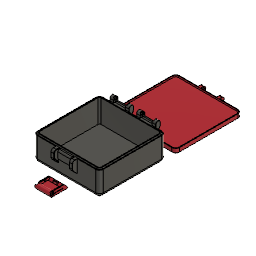
Milwaukee Tool Box Single Lock (Autodesk Fusion 360 design; units mm, degrees)
part number: 2025-08-27-12-33-30-467
Autodesk Fusion 360 part; units mm, degrees
sketch "Box" plane through (0, 0, 0) normal (0, 0, 1) x (1, 0, 0)
  line L0 (38, 43) -> (-38, 43)
  line L1 (-43, 38) -> (-43, -38)
  line L2 (-38, -43) -> (38, -43)
  line L3 (43, -38) -> (43, 38)
  line L4 (43, 43) -> (-43, -43) construction
  line L5 (-43, 43) -> (43, -43) construction
  arc A0 (-38, 43) -> (-43, 38) centre (-38, 38) ccw
  arc A1 (43, 38) -> (38, 43) centre (38, 38) ccw
  arc A2 (38, -43) -> (43, -38) centre (38, -38) ccw
  arc A3 (-43, -38) -> (-38, -43) centre (-38, -38) ccw
  line L6 (38, 40) -> (-38, 40)
  arc A4 (-38, 40) -> (-40, 38) centre (-38, 38) ccw
  line L7 (-40, 38) -> (-40, -38)
  arc A5 (-40, -38) -> (-38, -40) centre (-38, -38) ccw
  line L8 (-38, -40) -> (38, -40)
  arc A6 (38, -40) -> (40, -38) centre (38, -38) ccw
  line L9 (40, -38) -> (40, 38)
  arc A7 (40, 38) -> (38, 40) centre (38, 38) ccw
  line L10 (-41, 38) -> (-41, -38)
  arc A8 (-41, -38) -> (-38, -41) centre (-38, -38) ccw
  line L11 (-38, -41) -> (38, -41)
  arc A9 (38, -41) -> (41, -38) centre (38, -38) ccw
  line L12 (41, -38) -> (41, 38)
  arc A10 (41, 38) -> (38, 41) centre (38, 38) ccw
  line L13 (38, 41) -> (-38, 41)
  arc A11 (-38, 41) -> (-41, 38) centre (-38, 38) ccw
  dimension "d5" = 86
  dimension "d6" = 86
  dimension "d7" = 5
  dimension "d10" = -3
  dimension "d95" = 1
  constraint horizontal L0
  constraint perpendicular L0 L1
  constraint parallel L0 L2
  constraint parallel L1 L3
  constraint coincident L4 origin
  constraint coincident L5 origin
  constraint coincident L5.start L0
  constraint coincident L5.start L1
  constraint tangent L0 A0
  constraint tangent L1 A0
  constraint coincident L4.start L0
  constraint coincident L4.start L3
  constraint tangent L0 A1
  constraint tangent L3 A1
  constraint coincident L5.end L3
  constraint coincident L5.end L2
  constraint tangent L3 A2
  constraint tangent L2 A2
  constraint equal A1 A2
  constraint coincident L4.end L2
  constraint coincident L4.end L1
  constraint tangent L2 A3
  constraint tangent L1 A3
  constraint equal A0 A1
  constraint equal A0 A3
  measures "d5" distance of L4.end L5.end
  measures "d6" distance of L5.start L4.end
  measures "d7" radius of A0
extrude "Extrude1" add sketch "Box" along normal blind 31 contours L0 L1 L2 L3 A0 A1 A2 A3 makes body 1
extrude "Extrude15" add sketch "Box" along normal blind 32 contours L10 A8 L11 A9 L12 A10 L13 A11 bodies 1
extrude "Extrude2" add sketch "Box" along normal blind 2 contours L6 A4 L7 A5 L8 A6 L9 A7 bodies 1
chamfer "Chamfer7" distance 0.99 angle 45 8 edges at (0, -41, 31) (-40.1213, -40.1213, 31) (-41, 0, 31) (-40.1213, 40.1213, 31) (0, 41, 31) (40.1213, 40.1213, 31) (41, 0, 31) (40.1213, -40.1213, 31) on bodies 1
chamfer "Chamfer1" distance 3 angle 45 8 edges at (0, -43, 0) (41.5355, -41.5355, 0) (43, 0, 0) (41.5355, 41.5355, 0) (0, 43, 0) (-41.5355, 41.5355, 0) (-43, 0, 0) (-41.5355, -41.5355, 0) on bodies 1
fillet "Fillet1" radius 4 8 edges at (-41.5355, 41.5355, 3) (0, 43, 3) (41.5355, 41.5355, 3) (43, 0, 3) (41.5355, -41.5355, 3) (0, -43, 3) (-41.5355, -41.5355, 3) (-43, 0, 3) on bodies 1
sketch "Lid" plane through (0, 0, 31) normal (0, 0, 1) x (-1, 0, 0)
  arc A0 (43, 38) -> (38, 43) centre (38, 38) ccw
  line L0 (38, 43) -> (-38, 43)
  arc A1 (-38, 43) -> (-43, 38) centre (-38, 38) ccw
  line L1 (-43, 38) -> (-43, -38)
  arc A2 (-43, -38) -> (-38, -43) centre (-38, -38) ccw
  line L2 (-38, -43) -> (38, -43)
  arc A3 (38, -43) -> (43, -38) centre (38, -38) ccw
  line L3 (43, -38) -> (43, 38)
  arc A4 (38, -43) -> (43, -38) centre (38, -38) ccw
  line L4 (-38, -43) -> (38, -43)
  line L5 (43, -38) -> (43, 38)
  arc A5 (43, 38) -> (38, 43) centre (38, 38) ccw
  line L6 (38, 43) -> (-38, 43)
  arc A6 (-38, 43) -> (-43, 38) centre (-38, 38) ccw
  line L7 (-43, 38) -> (-43, -38)
  arc A7 (-43, -38) -> (-38, -43) centre (-38, -38) ccw
  line L8 (42.1, -38) -> (42.1, 38)
  arc A8 (42.1, 38) -> (38, 42.1) centre (38, 38) ccw
  line L9 (38, 42.1) -> (-38, 42.1)
  arc A9 (-38, 42.1) -> (-42.1, 38) centre (-38, 38) ccw
  line L10 (-42.1, 38) -> (-42.1, -38)
  arc A10 (-42.1, -38) -> (-38, -42.1) centre (-38, -38) ccw
  line L11 (-38, -42.1) -> (38, -42.1)
  arc A11 (38, -42.1) -> (42.1, -38) centre (38, -38) ccw
  arc A12 (-41.99, -38) -> (-38, -41.99) centre (-38, -38) ccw
  dimension "d18" = -0.9
extrude "Extrude3" add sketch "Lid" along normal blind 6 separate body contours A0 L0 A1 L1 A2 L2 A3 L3 A4 L4 L5 A5 L6 A6 L7 A7 | L8 A8 L9 A9 L10 A10 L11 A11 makes body 2
extrude "Extrude16" cut sketch "Lid" along normal blind 1 contours L8 A8 L9 A9 L10 A10 L11 A11 bodies 2
chamfer "Chamfer8" distance 1 angle 45 16 edges at (-40.8991, 40.8991, 32) (-42.1, 0, 32) (-40.8991, -40.8991, 32) (0, -42.1, 32) (40.8991, -40.8991, 32) (42.1, 0, 32) (40.8991, 40.8991, 32) (0, 42.1, 32) (0, -43, 37) (41.5355, -41.5355, 37) (43, 0, 37) (41.5355, 41.5355, 37) (0, 43, 37) (-41.5355, 41.5355, 37) (-43, 0, 37) (-41.5355, -41.5355, 37) on bodies 2
sketch "Lid Hinge and Latch" plane through (0, 0, 0) normal (1, 0, 0) x (0, 1, 0)
  circle A0 centre (46.2, 34) radius 1.8
  line L0 (43, 31) -> (46.2, 31)
  circle A1 centre (-46.2, 34) radius 1.8 construction
  line L1 (-44.8771, 32.5) -> (-43.9639, 32)
  circle A2 centre (-46.2, 34) radius 2
  circle A3 centre (-46.2, 34) radius 3
  line L2 (-44.8771, 35.5) -> (-43.9639, 36)
  line L3 (-49.2, 34) -> (-49.2, 14)
  line L4 (-49.2, 14) -> (-47.7, 14)
  line L5 (-47.7, 14) -> (-43, 18.7)
  line L6 (-43, 18.7) -> (-43, 31.4722)
  line L7 (-46.5, 31.015) -> (-46.5, 20.7)
  line L8 (-46.5, 20.7) -> (-43.5, 20.7)
  line L9 (-46, 20.7) -> (-46, 31.0067)
  line L10 (-43.9639, 32) -> (-43, 31.4722)
  line L11 (-43.5, 20.7) -> (-43, 20.2)
  line L12 (-46.5, 20.7) -> (-43.75, 17.95)
  line L13 (43, 31) -> (43, 36)
  line L14 (-43, 4.6569) -> (-43, 31)
  line L15 (43, 4.6569) -> (43, 31)
  line L16 (-49.2, 34) -> (-49.2, 35.2426)
  line L17 (-49.2, 35.2426) -> (-48.3213, 36.1213)
  line L18 (-38, 0) -> (-40, 0)
  line L19 (42, 37) -> (47, 37)
  line L20 (47, 37) -> (47.6938, 36.6017)
  line L21 (43, 36) -> (42, 37)
  circle A4 centre (46.2, 34) radius 3
  line L22 (-43, 31) -> (-43, 36)
  point P0 (-43, 31.4722)
  point P1 (-38, 0)
  point P2 (42, 37)
  dimension "d37" = 3.6
  dimension "d110" = 3.6
  dimension "d111" = 6
  dimension "d112" = 4
  dimension "d113" = 4
  dimension "d114" = 3
  dimension "d120" = 45
  dimension "d121" = 1.5
  dimension "d124" = 3
  dimension "d130" = 0.5
  dimension "d131" = 2
  dimension "d132" = 45
  dimension "d133" = 0.5
  dimension "d277" = 1.2426
  dimension "d337" = 89.2
  dimension "d342" = 34
  dimension "d343" = 14
  dimension "d353" = 5
  dimension "d354" = 29.863
  dimension "d355" = 6
  dimension "d356" = 89.2
  constraint coincident L1.end A3
  constraint coincident L2.end A3
  constraint concentric A1 A2
  constraint coincident L1.start A2
  constraint coincident A1.centre A2.centre
  constraint coincident L2.start A2
  constraint vertical L1.start L2.start
  constraint vertical L2.end L1.end
  constraint vertical L3
  constraint tangent A3 L3
  constraint perpendicular L3 L4
  constraint perpendicular L4 L6
  constraint vertical L7
  constraint vertical L9
  constraint parallel L1 L10
  constraint coincident A3 L7.start
  constraint coincident A3 L9.end
  constraint horizontal L8
  constraint coincident L9.start L8
  constraint coincident L6 L11.end
  constraint coincident L5 L12.end
  constraint perpendicular L5 L12
  constraint coincident A3 L3.start
  constraint coincident P0 L6.end
  constraint coincident P0 L14
  constraint coincident L0.start L13.start
  constraint perpendicular L0 L13
  constraint parallel L3 L16
  constraint coincident A3 L17.end
  constraint coincident L3.start L16.start
  constraint tangent A3 L17
  constraint horizontal L19
  constraint coincident P2 L19.start
  constraint concentric A0 A4
  constraint coincident L0.end A4
  constraint tangent L0 A4
  constraint coincident L20.end A4
  constraint tangent L20 A4
  measures "d37" diameter of A0
  measures "d110" diameter of A1
  measures "d111" diameter of A3
  measures "d112" distance of L2.end L1.end
  measures "d113" diameter of A2
  measures "d114" distance of L1.start L2.start
  measures "d120" angle of L4 L5
  measures "d121" distance of L3.end L4.end
  measures "d124" distance of L6 L9
  measures "d130" distance of L7.end L9.start
  measures "d131" distance of L5.end L8
  measures "d132" angle of L6 L11
  measures "d133" distance of L6 L8.end
  measures "d277" distance of L3.start L16.end
  measures "d337" distance of A1.centre L15
  measures "d342" distance of A1.centre L18
  measures "d343" distance of L4 L18
  measures "d353" distance of P2 L19.end
  measures "d354" angle of L19 L20
  measures "d355" diameter of A4
  measures "d356" distance of A0.centre L22
extrude "Extrude7" add sketch "Lid Hinge and Latch" along normal mid plane 15 from surface at 17.3333 separate body contours L0 L13 L19 L21 A4 | A4 | L19 L20 A4 makes body 3
extrude "Extrude8" add sketch "Lid Hinge and Latch" along normal mid plane 18 from surface at 17.3333 contours A0 bodies 3
chamfer "Chamfer2" distance 0.5 angle 45 2 faces at (8.3333, 46.7552, 33.4017) (26.3333, 46.7552, 33.4017) on bodies 3
sketch "Lid Hinge Cut" plane through (0, 43, 0) normal (0, 1, 0) x (-1, 0, 0)
  line L0 (-38, 31) -> (38, 31)
  line L1 (38, 31) -> (38, 36)
  line L2 (-38, 36) -> (-38, 31)
  line L3 (-24.8333, 35.8) -> (-26.3333, 34.934) construction
  line L4 (-26.3333, 34.934) -> (-26.3333, 35.8) construction
  line L5 (-26.3333, 35.8) -> (-24.8333, 35.8) construction
  line L6 (-9.8333, 35.8) -> (-8.3333, 34.934) construction
  line L7 (-8.3333, 34.934) -> (-8.3333, 35.8) construction
  line L8 (-8.3333, 35.8) -> (-9.8333, 35.8) construction
  line L9 (-25.8333, 35.8) -> (-25.8333, 32.2)
  line L10 (-8.8333, 32.2) -> (-8.8333, 35.8)
  line L11 (-26.3333, 32.7) -> (-26.3333, 35.3)
  line L12 (-8.3333, 35.3) -> (-8.3333, 32.7)
  line L13 (38, 36) -> (-38, 36)
  line L14 (-9.8333, 31) -> (-9.8333, 36)
  line L15 (-24.8333, 36) -> (-24.8333, 31)
  line L16 (-19.8333, 37) -> (-14.8333, 37)
  line L17 (-14.8333, 37) -> (-14.8333, 31)
  line L18 (-14.8333, 31) -> (-19.8333, 31)
  line L19 (-19.8333, 31) -> (-19.8333, 37)
  line L20 (-9.8333, 37) -> (-24.8333, 37)
  dimension "d357" = 30
  dimension "d358" = 30
  dimension "d365" = 5
  dimension "d366" = 5
  constraint perpendicular L0 L4
  constraint perpendicular L4 L5
  constraint perpendicular L0 L7
  constraint perpendicular L7 L8
  constraint coincident L3.end L11
  constraint coincident L6.end L12
  constraint coincident L3.start L15
  constraint coincident L6.start L14
  constraint coincident L5 L9.start
  constraint coincident L8 L10.end
  constraint horizontal L16
  constraint vertical L17
  constraint horizontal L18
  constraint vertical L19
  constraint coincident L0 L17.end
  constraint coincident L16.start L20
  measures "d357" angle of L3 L5
  measures "d358" angle of L6 L8
  measures "d365" distance of L17 L20.start
  measures "d366" distance of L16.start L20.end
extrude "Extrude40" cut sketch "Lid Hinge Cut" along normal through all contours L0 L13 L17 L18 L19 | L13 L16 L17 L19 L20 bodies 3
extrude "Extrude26" add sketch "Lid Hinge and Latch" along normal mid plane 20 separate body contours L1 A2 A3 L2 | A3 L6 L8 L9 L10 L11 L14 L22 | A3 L3 L4 L5 L7 L12 | L5 L6 L8 L11 L12 L14 | A3 L16 L17 picked at (-44.3747, 35.9359) makes body 4
extrude "Extrude27" add sketch "Lid Hinge and Latch" along normal mid plane 17 contours A2 bodies 4
extrude "Extrude28" add sketch "Lid Hinge and Latch" along normal mid plane 18 contours L1 A2 A3 L2 picked at (-44.1133, 35.6507) bodies 4
chamfer "Chamfer14" distance 0.49 angle 45 2 edges at (8.5, -48.0647, 34.7232) (-8.5, -48.0647, 34.7232) on bodies 4
chamfer "Chamfer15" distance 0.5 angle 45 2 edges at (9, -43.2, 34) (-9, -43.2, 34) on bodies 4
extrude "Extrude29" cut sketch "Lid Hinge and Latch" along normal mid plane 17 contours A3 L6 L8 L9 L10 L11 L14 L22 | L5 L6 L8 L11 L12 L14 bodies 4
extrude "Extrude30" add sketch "Lid Hinge and Latch" along normal mid plane 5 contours L5 L6 L8 L11 L12 L14 bodies 4
chamfer "Chamfer18" distance 0.4 angle 45 3 edges at (8.5, -43, 25.0861) (-8.5, -43, 25.0861) (0, -49.2, 14) on bodies 4
fillet "Fillet4" radius 1 1 edges at (0, -47.7, 14) on bodies 4
sketch "Box and Lacth Hinge" plane through (0, 0, 0) normal (1, 0, 0) x (0, 1, 0)
  line L0 (43, 31) -> (43, 23)
  line L1 (-46.2, 37) -> (-42, 37)
  line L2 (-46, 29) -> (-46, 21.2)
  line L3 (-45.5, 20.7) -> (-43, 20.7)
  line L4 (-43, 14) -> (-43, 31)
  line L5 (-46, 21.2) -> (-45.5, 20.7)
  arc A0 (-46.2, 31) -> (-49.2, 28) centre (-46.2, 28) ccw
  line L6 (-49.2, 28) -> (-49.2, 21.8569)
  line L7 (-48.0284, 19.0284) -> (-43, 14)
  line L8 (-45.5, 20.7) -> (-43, 18.2)
  line L9 (43.2, 31) -> (43.2, 34)
  line L10 (48.0284, 28.0284) -> (43, 23)
  arc A1 (-49.2, 21.8569) -> (-48.0284, 19.0284) centre (-45.2, 21.8569) ccw
  circle A2 centre (-46.2, 34) radius 3
  line L11 (-43, 31) -> (-46.2, 31)
  arc A3 (-44, 31) -> (-46, 29) centre (-44, 29) ccw
  line L12 (43, 31) -> (45.0864, 31)
  line L13 (-43, 31) -> (-43, 36)
  circle A4 centre (-46.2, 34) radius 1.8
  arc A5 (48.0284, 28.0284) -> (49.2, 30.8569) centre (45.2, 30.8569) ccw
  line L14 (49.2, 34) -> (49.2, 30.8569)
  circle A6 centre (46.2, 34) radius 2
  circle A7 centre (46.2, 34) radius 1.8 construction
  circle A8 centre (46.2, 34) radius 3
  line L15 (47.7, 35.3229) -> (48.2, 36.2361)
  line L16 (44.7, 35.3229) -> (44.2, 36.2361)
  circle A9 centre (46.2, 34) radius 3.2 construction
  line L17 (43, 31) -> (46.2, 31)
  line L18 (-38, 0) -> (38, 0)
  line L19 (-43, 36) -> (-42, 37)
  line L20 (-46.2, 37) -> (-47, 37)
  line L21 (-47, 37) -> (-47.6938, 36.6017)
  circle A10 centre (46.2, 34) radius 1.3
  line L22 (47.3136, 31) -> (49.2, 31)
  arc A11 (45.0864, 31) -> (47.3136, 31) centre (46.2, 34) ccw
  point P0 (-46, 20.7)
  point P1 (-46, 20.7)
  point P2 (-49.2, 34)
  point P3 (-48.8, 14)
  point P4 (43, 31)
  point P5 (43, 31)
  point P6 (43, 36)
  dimension "d136" = 0.5
  dimension "d137" = 0.5
  dimension "d140" = 3
  dimension "d150" = 45
  dimension "d182" = 45
  dimension "d239" = 4
  dimension "d244" = 3
  dimension "d252" = 2
  dimension "d270" = 4
  dimension "d309" = 3.6
  dimension "d310" = 6
  dimension "d311" = 4
  dimension "d312" = 4
  dimension "d313" = 3
  dimension "d321" = 6.4
  dimension "d352" = 23
  dimension "d363" = 0.8
  constraint vertical L2
  constraint horizontal L3
  constraint vertical L4
  constraint coincident P1 L2
  constraint coincident P1 L3
  constraint horizontal A0.end A0.centre
  constraint vertical L6
  constraint parallel L5 L8
  constraint coincident L4 L3.end
  constraint vertical L9
  constraint coincident L0.end L10.end
  constraint vertical L0
  constraint tangent L6 A1
  constraint tangent L7 A1
  constraint coincident A2 A0.start
  constraint tangent A2 L11
  constraint horizontal L11
  constraint coincident L11 A3.start
  constraint tangent L2 A3
  constraint tangent L11 A3
  constraint coincident P1 P0
  constraint coincident L4 L8.end
  constraint vertical A0.end P2
  constraint coincident L1.start A2
  constraint horizontal L1
  constraint horizontal L4.start P3
  constraint horizontal L12
  constraint coincident P5 P4
  constraint coincident L12 A11.start
  constraint tangent L10 A5
  constraint vertical L14
  constraint coincident A5.end L14.end
  constraint tangent A5 L14
  constraint coincident L15.end A8
  constraint coincident L16.end A8
  constraint concentric A6 A7
  constraint coincident L15.start A6
  constraint coincident L16.start A6
  constraint coincident L9.end A8
  constraint horizontal L9.end A6.centre
  constraint coincident L14.start A8
  constraint concentric A8 A9
  constraint horizontal L14.start A6.centre
  constraint horizontal L15.start L16.start
  constraint horizontal L16.end L15.end
  constraint vertical L1.start A2.centre
  constraint coincident A6.centre A7.centre
  constraint coincident L12 L9.start
  constraint tangent A2 L20
  constraint coincident A2 L21.end
  constraint tangent A2 L21
  constraint coincident L1.end L19.end
  constraint coincident A9 L22.start
  constraint coincident L14 L22.end
  constraint perpendicular L14 L22
  constraint horizontal L12.end L22.start
  constraint coincident L12.end A9
  constraint concentric A9 A11
  measures "d136" distance of P1 L2.end
  measures "d137" distance of P1 L3.start
  measures "d140" distance of L2 L4
  measures "d150" angle of L4 L7
  measures "d182" angle of L0 L10
  measures "d239" radius of A1
  measures "d244" radius of A0
  measures "d252" radius of A3
  measures "d270" radius of A5
  measures "d309" diameter of A7
  measures "d310" diameter of A8
  measures "d311" distance of L16.end L15.end
  measures "d312" diameter of A6
  measures "d313" distance of L15.start L16.start
  measures "d321" diameter of A9
  measures "d352" distance of L0.end L18
  measures "d363" distance of L1.start L20.end
extrude "Extrude11" add sketch "Box and Lacth Hinge" along normal mid plane 25 from surface at 17.3333 separate body contours L0 L10 L12 A5 L14 L17 L22 A11 | L9 L12 A8 L17 | A6 A8 L15 L16 | L14 A8 L17 L22 A11 | A6 A8 L15 L16 | A6 | A10 makes body 5
extrude "Extrude10" cut sketch "Box and Lacth Hinge" along normal mid plane 15.4 from surface at 17.3333 contours L9 L12 A8 L17 | A6 A8 L15 L16 | L14 A8 L17 L22 A11 | A6 A8 L15 L16 | L1 A2 L11 L13 L19 bodies 5
extrude "Extrude12" cut sketch "Box and Lacth Hinge" along normal mid plane 18.4 from surface at 17.3333 contours A6 | A10 bodies 5
extrude "Extrude39" cut sketch "Box and Lacth Hinge" along normal mid plane 17.4 from surface at 17.3333 contours A6 A8 L15 L16 picked at (44.5493, 36.0867) bodies 5
chamfer "Chamfer4" distance 0.499 angle 45 2 faces at (8.1333, 45.0225, 34.3325) (26.5333, 45.0225, 33.754) on bodies 5
chamfer "Chamfer21" distance 0.5 distance2 0.5 2 edges at (8.6333, 46.2, 37) (26.0333, 46.2, 37) measured on face at (6.4333, 43.8719, 35.892) measured on face at (28.2333, 43.8719, 35.892) on bodies 5
chamfer "Chamfer3" distance 0.2 angle 45 10 edges at (4.8333, 46.2, 37) (4.8333, 49.2, 32.4284) (4.8333, 48.8955, 29.3261) (4.8333, 45.5142, 25.5142) (4.8333, 43.2, 32.5) (29.8333, 49.2, 32.4284) (29.8333, 46.2, 37) (29.8333, 43.2, 32.5) (29.8333, 45.5142, 25.5142) (29.8333, 48.8955, 29.3261) on bodies 5
extrude "Extrude31" add sketch "Box and Lacth Hinge" along normal mid plane 28 contours L1 A2 L11 L13 L19 | A2 | A2 L20 L21 | A4 bodies 2
extrude "Extrude32" cut sketch "Box and Lacth Hinge" along normal mid plane 20.4 contours L1 A2 L11 L13 L19 | A2 | A2 L20 L21 bodies 2
extrude "Extrude33" cut sketch "Box and Lacth Hinge" along normal mid plane 17.4 contours A4 bodies 2
chamfer "Chamfer17" distance 0.5 angle 45 2 edges at (8.7, -47.8782, 33.3491) (-8.7, -47.8782, 34.6509) on bodies 2
chamfer "Chamfer16" distance 0.2 angle 45 6 edges at (14, -49.0987, 33.227) (14, -47.3469, 36.8008) (14, -44.6, 31) (-14, -49.0987, 33.227) (-14, -44.6, 31) (-14, -47.3469, 36.8008) on bodies 2
extrude "Extrude21" add sketch "Box and Lacth Hinge" along normal mid plane 28 separate body contours L2 L4 L5 A0 L6 L7 L8 A1 L11 A3 | L2 L3 L4 L5 L11 A3 | L3 L4 L8 makes body 6
extrude "Extrude22" cut sketch "Box and Lacth Hinge" along normal mid plane 20.4 contours L2 L4 L5 A0 L6 L7 L8 A1 L11 A3 | L2 L3 L4 L5 L11 A3 | L3 L4 L8 bodies 6 makes body 7 at (14, -44.6761, 21.3428)
chamfer "Chamfer11" distance 0.2 angle 45 10 edges at (-14, -49.2, 24.9284) (-14, -48.3213, 30.1213) (-14, -44.6, 31) (-14, -45.5142, 16.5142) (-14, -48.8955, 20.3261) (14, -49.2, 24.9284) (14, -48.8955, 20.3261) (14, -45.5142, 16.5142) (14, -44.6, 31) (14, -48.3213, 30.1213) on bodies 6 7
sketch "Latch Side" plane through (0, 0, 0) normal (1, 0, 0) x (0, 1, 0)
  line L0 (-48.0284, 19.0284) -> (-43, 14)
  line L1 (-43, 14) -> (-43, 31)
  arc A0 (-46.2, 31) -> (-49.2, 28) centre (-46.2, 28) ccw
  line L2 (-49.2, 28) -> (-49.2, 21.8569)
  arc A1 (-49.2, 21.8569) -> (-48.0284, 19.0284) centre (-45.2, 21.8569) ccw
  line L3 (-43, 31) -> (-46.2, 31)
  line L4 (-43, 30) -> (-46.2, 30)
  arc A2 (-46.2, 30) -> (-48.2, 28) centre (-46.2, 28) ccw
  line L5 (-48.2, 28) -> (-48.2, 21.8569)
  arc A3 (-48.2, 21.8569) -> (-47.3213, 19.7355) centre (-45.2, 21.8569) ccw
  line L6 (-47.3213, 19.7355) -> (-43, 15.4142)
  dimension "d224" = -1
  constraint coincident L1 L6.end
  constraint coincident L1 L4.start
extrude "Extrude25" cut sketch "Latch Side" along normal mid plane 21.4 contours L1 L4 A2 L5 A3 L6 bodies 6 7
chamfer "Chamfer13" distance 0.49 angle 45 10 edges at (-10.7, -44.6, 30) (-10.7, -45.1607, 17.5749) (-10.7, -47.9716, 20.7088) (-10.7, -48.2, 24.9284) (-10.7, -47.6142, 29.4142) (10.7, -47.6142, 29.4142) (10.7, -48.2, 24.9284) (10.7, -47.9716, 20.7088) (10.7, -45.1607, 17.5749) (10.7, -44.6, 30) on bodies 6 7
extrude "Extrude19" add sketch "Box and Lacth Hinge" along normal mid plane 16.6 separate body contours L2 L3 L4 L5 L11 A3 | L3 L4 L8 makes body 8
extrude "Extrude20" cut sketch "Box and Lacth Hinge" along normal mid plane 5.6 contours L3 L4 L8 bodies 8
ref_plane "WorkPlane1" through (0, -44.5, 24.6) normal (0, 1, 0) x (0, 0, 1)
sketch "Nub" plane through (0, -44.5, 0) normal (0, 1, 0) x (1, 0, 0)
  line L0 (-8.3, -25.1) -> (8.3, -25.1)
  line L1 (-8.3, -21.2) -> (-8.3, -29)
  line L2 (8.3, -29) -> (8.3, -21.2)
  line L3 (-8.3, -25.1) -> (-8.9, -25.1)
  line L4 (-7.9, -26.1) -> (7.9, -26.1)
  line L5 (8.3, -25.1) -> (8.9, -25.1)
  line L6 (-8.9, -25.1) -> (8.9, -25.1)
  arc A0 (-8.9, -25.1) -> (-7.9, -26.1) centre (-7.9, -25.1) ccw
  arc A1 (7.9, -26.1) -> (8.9, -25.1) centre (7.9, -25.1) ccw
  arc A2 (-9.015, -25.1) -> (-7.9, -26.215) centre (-7.9, -25.1) ccw
  line L7 (-7.9, -26.215) -> (7.9, -26.215)
  arc A3 (7.9, -26.215) -> (9.015, -25.1) centre (7.9, -25.1) ccw
  line L8 (-9.015, -25.1) -> (-8.9, -25.1)
  line L9 (8.9, -25.1) -> (9.015, -25.1)
  point P0 (0, -25.1)
  dimension "d176" = 1
  dimension "d225" = 16.6
  dimension "d226" = 17.8
  dimension "d228" = 1
  dimension "d229" = 1
  dimension "d231" = 0.115
  constraint horizontal L0
  constraint coincident L0.end L2
  constraint midpoint L0.start L1
  constraint perpendicular L1 L3
  constraint perpendicular L2 L4
  constraint horizontal L5
  constraint equal L3 L5
  constraint midpoint L0 P0
  constraint midpoint P0 L6
  constraint tangent L4 A0
  constraint coincident L3.end L6.start
  constraint tangent L4 A1
  constraint parallel L3 L8
  constraint parallel L5 L9
  measures "d176" distance of L0 L4
  measures "d225" distance of L0.start L0.end
  measures "d226" distance of L3.end L5.end
  measures "d228" radius of A0
  measures "d229" radius of A1
revolve "Revolve1" add sketch "Nub" angle 360 about axis through (-8.3, -44.5, 25.1) along (1, 0, 0) contours L0 L1 L2 L4 L6 A0 A1 | L1 L3 L6 A0 | L2 L5 L6 A1 bodies 8
revolve "Revolve2" cut sketch "Nub" angle 360 about axis through (-8.3, -44.5, 25.1) along (1, 0, 0) contours L1 L3 L6 A0 | L2 L5 L6 A1 | L1 A0 A2 L8 | L2 A1 A3 L9 bodies 4
mirror "Mirror8" about plane through (0, 0, 0) normal (1, 0, 0) of bodies 3 5 makes body 9 at (-13.2333, 43, 28.3333) makes body 10 at (-23.1667, 44, 37)
combine "Combine8" operation add target body 2 tool bodies 3 10
combine "Combine9" operation add target body 1 tool bodies 6 7 5 9 8
sketch "Column Divider" plane through (0, 0, 2) normal (0, 0, 1) x (-1, 0, 0)
  arc A0 (-40, -38) -> (-38, -40) centre (-38, -38) ccw
  line L0 (-38, -40) -> (38, -40)
  arc A1 (38, -40) -> (40, -38) centre (38, -38) ccw
  line L1 (40, -38) -> (40, 38)
  arc A2 (40, 38) -> (38, 40) centre (38, 38) ccw
  line L2 (38, 40) -> (-38, 40)
  arc A3 (-38, 40) -> (-40, 38) centre (-38, 38) ccw
  line L3 (-40, 38) -> (-40, -38)
  line L4 (41, -41) -> (41, 41)
  line L5 (40, 1) -> (42, 1)
  line L6 (42, 1) -> (42, -1)
  line L7 (42, -1) -> (40, -1)
  line L8 (40, -1) -> (40, 1)
  line L9 (40, 1) -> (42, -1) construction
  line L10 (42, 1) -> (40, -1) construction
  point P0 (38, 41)
  point P1 (41, 38)
  point P2 (38, -41)
  point P3 (41, -38)
  point P4 (41, 0)
  dimension "d344" = 2
  dimension "d345" = 2
  constraint vertical L4
  constraint horizontal L4.start P2
  constraint horizontal L4.end P0
  constraint coincident L4 P1
  constraint horizontal L5
  constraint perpendicular L5 L6
  constraint parallel L5 L7
  constraint parallel L6 L8
  constraint coincident L9 P4
  constraint coincident L10 P4
  constraint midpoint L4 P4
  measures "d344" distance of L6.end L7.end
  measures "d345" distance of L5.end L6.end
extrude "Extrude35" add sketch "Column Divider" along normal blind 30 thin wall 2 centred separate body open curves L4 makes body 11
extrude "Extrude41" add sketch "Column Divider" against normal blind 2 contours L1 L4 L5 L7 L8 | L4 L5 L6 L7 bodies 11
pattern_linear "R-Pattern1" count 1 spacing 82 along (1, 0, 0) of bodies 11 merged
delete_body "RemoveBody1" bodies 11
sketch "Row Divider" plane through (0, 0, 2) normal (0, 0, 1) x (-1, 0, 0)
  arc A0 (-40, -38) -> (-38, -40) centre (-38, -38) ccw
  line L0 (-38, -40) -> (38, -40)
  arc A1 (38, -40) -> (40, -38) centre (38, -38) ccw
  line L1 (40, -38) -> (40, 38)
  arc A2 (40, 38) -> (38, 40) centre (38, 38) ccw
  line L2 (38, 40) -> (-38, 40)
  arc A3 (-38, 40) -> (-40, 38) centre (-38, 38) ccw
  line L3 (-40, 38) -> (-40, -38)
  line L4 (41, 41) -> (-41, 41)
  line L5 (-1, 42) -> (1, 42)
  line L6 (1, 42) -> (1, 40)
  line L7 (1, 40) -> (-1, 40)
  line L8 (-1, 40) -> (-1, 42)
  line L9 (-1, 42) -> (1, 40) construction
  line L10 (1, 42) -> (-1, 40) construction
  point P0 (38, 41)
  point P1 (41, 38)
  point P2 (-41, 38)
  point P3 (0, 41)
  dimension "d348" = 2
  dimension "d349" = 2
  constraint horizontal L4
  constraint coincident L4 P0
  constraint vertical L4.start P1
  constraint vertical L4.end P2
  constraint horizontal L5
  constraint perpendicular L5 L6
  constraint parallel L5 L7
  constraint parallel L6 L8
  constraint coincident L9 P3
  constraint coincident L10 P3
  constraint midpoint L4 P3
  measures "d348" distance of L6.end L7.end
  measures "d349" distance of L5.end L6.end
extrude "Extrude36" add sketch "Row Divider" along normal blind 30 thin wall 2 centred separate body open curves L4 makes body 12
extrude "Extrude42" add sketch "Row Divider" against normal blind 2 contours L2 L4 L6 L7 L8 | L4 L5 L6 L8 bodies 12
pattern_linear "R-Pattern2" count 1 spacing 82 along (0, 1, 0) of bodies 12 merged
delete_body "RemoveBody2" bodies 12
sketch "Sketch20" plane through (0, 0, 37) normal (0, 0, 1) x (-1, 0, 0)
  line L0 (-14, 42) -> (-38, 42)
  arc A0 (-38, 42) -> (-42, 38) centre (-38, 38) ccw
  line L1 (-42, 38) -> (-42, -38)
  arc A1 (-42, -38) -> (-38, -42) centre (-38, -38) ccw
  arc A2 (38, -42) -> (42, -38) centre (38, -38) ccw
  line L2 (42, -38) -> (42, 38)
  arc A3 (42, 38) -> (38, 42) centre (38, 38) ccw
  line L3 (-25, -43) -> (25, -43) construction
  line L4 (25, -43) -> (25, 43) construction
  line L5 (25, 43) -> (-25, 43) construction
  line L6 (-25, 43) -> (-25, -43) construction
  line L7 (-25, -43) -> (25, 43) construction
  line L8 (25, -43) -> (-25, 43) construction
  line L9 (-26.1621, -4.1639) -> (-12.9321, 0.866)
  line L10 (-12.9321, 0.866) -> (-13.6937, -0.7988)
  line L11 (-13.6937, -0.7988) -> (4.2298, 5.3292)
  line L12 (4.2298, 5.3292) -> (3.238, 3.2747)
  line L13 (3.238, 3.2747) -> (24.0483, 11.2623)
  line L14 (24.0483, 11.2623) -> (8.4096, 7.3482)
  line L15 (8.4096, 7.3482) -> (9.7025, 9.8101)
  line L16 (9.7025, 9.8101) -> (-9.6733, 2.6017)
  line L17 (-9.6733, 2.6017) -> (-8.5752, 4.7447)
  line L18 (-8.5752, 4.7447) -> (-26.1621, -4.1639)
  line L19 (12.3768, -8.1134) -> (14.6615, -6.1829)
  spline S0 degree 2 poles (14.6615, -6.1829) (15.5648, -7.2101) (15.6533, -7.281) knots 0 0 0 1 1 1
  spline S1 degree 2 poles (15.6533, -7.281) (15.7242, -7.2101) (17.6015, -5.6162) knots 0 0 0 1 1 1
  line L20 (17.6015, -5.6162) -> (17.3359, -8.2551)
  line L21 (17.3359, -8.2551) -> (24.0483, -2.623)
  line L22 (24.0483, -2.623) -> (19.4612, -4.8192)
  line L23 (19.4612, -4.8192) -> (20.6301, 5.0635)
  spline S2 degree 2 poles (20.6301, 5.0635) (19.2309, 6.1085) (19.107, 6.1793) knots 0 0 0 1 1 1
  spline S3 degree 3 poles (19.107, 6.1793) (18.983, 5.2406) (17.8495, -3.8096) (17.7964, -4.3055) knots 0 0 0 0 1 1 1 1
  line L24 (17.7964, -4.3055) -> (17.7964, -4.3233)
  line L25 (17.7964, -4.3233) -> (16.468, -5.439)
  line L26 (16.468, -5.439) -> (16.1847, -5.1557)
  line L27 (16.1847, -5.1557) -> (17.2473, 3.8592)
  spline S4 degree 2 poles (17.2473, 3.8592) (15.8127, 4.9218) (15.7242, 4.9927) knots 0 0 0 1 1 1
  spline S5 degree 3 poles (15.7242, 4.9927) (15.7065, 4.9041) (14.7501, -3.2606) (14.5375, -5.2088) knots 0 0 0 0 1 1 1 1
  line L28 (14.5375, -5.2088) -> (13.2269, -6.3246)
  line L29 (13.2269, -6.3246) -> (12.9436, -6.0412)
  line L30 (12.9436, -6.0412) -> (13.9708, 2.7434)
  line L31 (13.9708, 2.7434) -> (12.4477, 3.8592)
  line L32 (12.4477, 3.8592) -> (11.2079, -6.8382)
  line L33 (11.2079, -6.8382) -> (12.3768, -8.1134)
  line L34 (8.6398, -6.1475) -> (10.2338, -5.8818)
  line L35 (10.2338, -5.8818) -> (10.4286, -4.3233)
  line L36 (10.4286, -4.3233) -> (8.8523, -4.6243)
  line L37 (8.8523, -4.6243) -> (8.6398, -6.1475)
  line L38 (0.1386, -5.4922) -> (0.7762, -0.5685)
  line L39 (0.7762, -0.5685) -> (1.1304, -0.1966)
  line L40 (1.1304, -0.1966) -> (1.7148, -0.6925)
  line L41 (1.7148, -0.6925) -> (1.1304, -5.3151)
  line L42 (1.1304, -5.3151) -> (2.7067, -4.9254)
  line L43 (2.7067, -4.9254) -> (3.3265, -0.1081)
  line L44 (3.3265, -0.1081) -> (3.787, 0.5118)
  line L45 (3.787, 0.5118) -> (4.2829, 0.069)
  line L46 (4.2829, 0.069) -> (3.6985, -4.7837)
  line L47 (3.6985, -4.7837) -> (5.2924, -4.4472)
  line L48 (5.2924, -4.4472) -> (5.8238, -0.0372)
  line L49 (5.8238, -0.0372) -> (6.4791, 0.866)
  line L50 (6.4791, 0.866) -> (6.9396, 0.4764)
  line L51 (6.9396, 0.4764) -> (5.9123, -7.8123)
  line L52 (5.9123, -7.8123) -> (7.4709, -7.5644)
  line L53 (7.4709, -7.5644) -> (8.4273, 0.4056)
  line L54 (8.4273, 0.4056) -> (9.2066, 1.4859)
  line L55 (9.2066, 1.4859) -> (9.6139, 1.1671)
  line L56 (9.6139, 1.1671) -> (8.9409, -3.6857)
  line L57 (8.9409, -3.6857) -> (10.5349, -3.3669)
  line L58 (10.5349, -3.3669) -> (11.261, 2.2652)
  line L59 (11.261, 2.2652) -> (9.8796, 3.3633)
  line L60 (9.8796, 3.3633) -> (8.4981, 1.5036)
  line L61 (8.4981, 1.5036) -> (7.0635, 2.6548)
  line L62 (7.0635, 2.6548) -> (5.6821, 0.7775)
  line L63 (5.6821, 0.7775) -> (4.1944, 2.0527)
  line L64 (4.1944, 2.0527) -> (2.7421, 0.1222)
  line L65 (2.7421, 0.1222) -> (1.5554, 1.1671)
  line L66 (1.5554, 1.1671) -> (-0.499, -1.0644)
  line L67 (-0.499, -1.0644) -> (-1.1366, -5.7756)
  line L68 (-1.1366, -5.7756) -> (0.1386, -5.4922)
  line L69 (-21.6281, -5.7047) -> (-21.1677, -6.0943)
  line L70 (-21.1677, -6.0943) -> (-21.2562, -6.8382)
  line L71 (-21.2562, -6.8382) -> (-23.3815, -8.0426)
  line L72 (-23.3815, -8.0426) -> (-21.6636, -10.1679)
  line L73 (-21.6636, -10.1679) -> (-20.0873, -8.8041)
  line L74 (-20.0873, -8.8041) -> (-19.7154, -5.8464)
  line L75 (-19.7154, -5.8464) -> (-17.6255, -4.6952)
  line L76 (-17.6255, -4.6952) -> (-17.1296, -5.1025)
  line L77 (-17.1296, -5.1025) -> (-17.2358, -5.8995)
  line L78 (-17.2358, -5.8995) -> (-19.556, -7.1747)
  line L79 (-19.556, -7.1747) -> (-17.714, -9.4417)
  line L80 (-17.714, -9.4417) -> (-16.0138, -7.9894)
  line L81 (-16.0138, -7.9894) -> (-15.6596, -5.1734)
  line L82 (-15.6596, -5.1734) -> (-14.898, -4.4472)
  line L83 (-14.898, -4.4472) -> (-13.7114, -6.8028)
  line L84 (-13.7114, -6.8028) -> (-16.368, -9.2292)
  line L85 (-16.368, -9.2292) -> (-15.1637, -9.0521)
  line L86 (-15.1637, -9.0521) -> (-13.1446, -7.3518)
  line L87 (-13.1446, -7.3518) -> (-13.6228, -11.1774)
  line L88 (-13.6228, -11.1774) -> (-12.1705, -10.9826)
  line L89 (-12.1705, -10.9826) -> (-11.3735, -4.4118)
  line L90 (-11.3735, -4.4118) -> (-10.488, -3.4377)
  line L91 (-10.488, -3.4377) -> (-10.2754, -3.6148)
  line L92 (-10.2754, -3.6148) -> (-10.8068, -7.7769)
  line L93 (-10.8068, -7.7769) -> (-9.2482, -7.4227)
  line L94 (-9.2482, -7.4227) -> (-8.7523, -3.6502)
  line L95 (-8.7523, -3.6502) -> (-8.0616, -2.8178)
  line L96 (-8.0616, -2.8178) -> (-7.7605, -3.0835)
  line L97 (-7.7605, -3.0835) -> (-8.2918, -7.2101)
  line L98 (-8.2918, -7.2101) -> (-6.7156, -6.8913)
  line L99 (-6.7156, -6.8913) -> (-6.2196, -3.0304)
  line L100 (-6.2196, -3.0304) -> (-5.4935, -2.1094)
  line L101 (-5.4935, -2.1094) -> (-5.1747, -2.3928)
  line L102 (-5.1747, -2.3928) -> (-5.7237, -6.7142)
  line L103 (-5.7237, -6.7142) -> (-4.1475, -6.3777)
  line L104 (-4.1475, -6.3777) -> (-4.112, -6.0412)
  line L105 (-4.112, -6.0412) -> (-3.014, -6.5725)
  line L106 (-3.014, -6.5725) -> (-1.4731, -4.6066)
  line L107 (-1.4731, -4.6066) -> (-1.0304, -1.0822)
  line L108 (-1.0304, -1.0822) -> (-2.5181, 0.193)
  line L109 (-2.5181, 0.193) -> (-3.8818, -1.5781)
  line L110 (-3.8818, -1.5781) -> (-5.0507, -0.5863)
  line L111 (-5.0507, -0.5863) -> (-6.3436, -2.2334)
  line L112 (-6.3436, -2.2334) -> (-7.4417, -1.2593)
  line L113 (-7.4417, -1.2593) -> (-8.646, -2.8533)
  line L114 (-8.646, -2.8533) -> (-9.7973, -1.8437)
  line L115 (-9.7973, -1.8437) -> (-11.3558, -3.544)
  line L116 (-11.3558, -3.544) -> (-12.5424, -2.6053)
  line L117 (-12.5424, -2.6053) -> (-12.8967, -5.4922)
  line L118 (-12.8967, -5.4922) -> (-14.1541, -2.9241)
  line L119 (-14.1541, -2.9241) -> (-15.819, -4.5358)
  line L120 (-15.819, -4.5358) -> (-16.8993, -3.6325)
  line L121 (-16.8993, -3.6325) -> (-20.105, -5.4036)
  line L122 (-20.105, -5.4036) -> (-20.9197, -4.6952)
  line L123 (-20.9197, -4.6952) -> (-23.8774, -6.4131)
  line L124 (-23.8774, -6.4131) -> (-23.966, -7.0507)
  line L125 (-23.966, -7.0507) -> (-21.6281, -5.7047)
  line L126 (-21.5396, -8.9458) -> (-22.2303, -8.1311)
  line L127 (-22.2303, -8.1311) -> (-21.3802, -7.6529)
  line L128 (-21.3802, -7.6529) -> (-21.5396, -8.9458)
  line L129 (-17.5546, -8.1311) -> (-18.2985, -7.2633)
  line L130 (-18.2985, -7.2633) -> (-17.3598, -6.7497)
  line L131 (-17.3598, -6.7497) -> (-17.5546, -8.1311)
  line L132 (-3.6161, -2.2511) -> (-2.9785, -1.4718)
  line L133 (-2.9785, -1.4718) -> (-2.642, -1.7729)
  line L134 (-2.642, -1.7729) -> (-3.1557, -5.8641)
  line L135 (-3.1557, -5.8641) -> (-4.0235, -5.4036)
  line L136 (-4.0235, -5.4036) -> (-3.6161, -2.2511)
  line L137 (10.2, 42) -> (-10.2, 42)
  line L138 (-24.8333, -42) -> (-24.8333, -47)
  line L139 (-24.8333, -47) -> (-19.8333, -47)
  line L140 (-19.8333, -47) -> (-19.8333, -43)
  line L141 (-19.8333, -43) -> (-14.8333, -43)
  line L142 (-14.8333, -43) -> (-14.8333, -47)
  line L143 (-14.8333, -47) -> (-9.8333, -47)
  line L144 (-9.8333, -47) -> (-9.8333, -42)
  line L145 (-38, -42) -> (-24.8333, -42)
  line L146 (9.8333, -42) -> (9.8333, -47)
  line L147 (9.8333, -47) -> (14.8333, -47)
  line L148 (14.8333, -47) -> (14.8333, -43)
  line L149 (14.8333, -43) -> (19.8333, -43)
  line L150 (19.8333, -43) -> (19.8333, -47)
  line L151 (19.8333, -47) -> (24.8333, -47)
  line L152 (24.8333, -47) -> (24.8333, -42)
  line L153 (38, 42) -> (14, 42)
  line L154 (14, 42) -> (10.2, 42)
  line L155 (-10.2, 42) -> (-14, 42)
  line L156 (-9.8333, -42) -> (9.8333, -42)
  line L157 (24.8333, -42) -> (38, -42)
  point P0 (-38, -43)
  dimension "d367" = 50
  constraint horizontal L3
  constraint perpendicular L3 L4
  constraint parallel L3 L5
  constraint parallel L4 L6
  constraint coincident L7 origin
  constraint coincident L8 origin
  constraint horizontal L3.start P0
  measures "d367" distance of L3.start L3.end
extrude "Extrude43" add sketch "Sketch20" against normal blind 0.6 separate body contours L9 L10 L11 L12 L13 L14 L15 L16 L17 L18 | L19 S0 S1 L20 L21 L22 L23 S2 S3 L24 L25 L26 L27 S4 S5 L28 L29 L30 L31 L32 L33 | L34 L35 L36 L37 | L38 L39 L40 L41 L42 L43 L44 L45 L46 L47 L48 L49 L50 L51 L52 L53 L54 L55 L56 L57 L58 L59 L60 L61 L62 L63 L64 L65 L66 L67 L68 | L69 L70 L71 L72 L73 L74 L75 L76 L77 L78 L79 L80 L81 L82 L83 L84 L85 L86 L87 L88 L89 L90 L91 L92 L93 L94 L95 L96 L97 L98 L99 L100 L101 L102 L103 L104 L105 L106 L107 L108 L109 L110 L111 L112 L113 L114 L115 L116 L117 L118 L119 L120 L121 L122 L123 L124 L125 makes body 13 at (-10.4699, -0.0218, 37) makes body 14 at (-9.8382, 4.9431, 37) makes body 15 at (4.974, 4.8369, 37) makes body 16 at (-19.2959, 1.3537, 37) makes body 17 at (-1.4197, -5.9137, 37)
scale "Scale1" factor 1 about (0, 0, 37) bodies 13 14 15 17 16
combine "Combine10" operation cut target body 2 tool bodies 13 14 15 17 16 keep tools
move_body "Move4" bodies 4 to x (1, 0, 0) y (0, 0, 1) z (0, -1, 0) at (0, -12.2, 80.2)
move_body "Move5" bodies 4 to x (1, 0, 0) y (0, 1, 0) z (0, 0, 1) at (0, -25, -31)
move_body "Move8" bodies 2 13 14 15 17 16 to x (1, 0, 0) y (0, -1, 0) z (0, 0, -1) at (0, 84, 74)
move_body "Move7" bodies 2 13 14 15 17 16 to x (1, 0, 0) y (0, 1, 0) z (0, 0, 1) at (0, 15, -37)
equation "Width = ( ( SlotWidth + 2 mm ) * Rows ) + 4 mm"
equation "Length = ( ( SlotLength + 2 mm ) * Columns ) + 4 mm"
equation "Height = SlotHeight + 8 mm"
equation "ConrnerRadius = 5 mm"
equation "d5 = Length"
equation "d6 = Width"
equation "d7 = ConrnerRadius"
equation "d11 = Height - 7 mm"
equation "HingePosition = ( HingesDistance / 2 ) + 14 mm"
equation "d46 = HingePosition"
equation "d47 = HingeSize"
equation "d49 = HingePosition"
equation "d50 = HingeSize + 3 mm"
equation "d61 = HingePosition"
equation "d62 = HingeSize + 0.4 mm"
equation "d64 = HingePosition"
equation "d65 = HingeSize + 10 mm"
equation "d67 = HingePosition"
equation "d68 = HingeSize + 3.4 mm"
equation "HingesDistance = ( Length - ( ConrnerRadius * 2 ) - 56 mm ) / 3"
equation "d97 = Height - 6 mm"
equation "d148 = LatchSize - 3.4 mm"
equation "d156 = LatchSize + 8 mm"
equation "d159 = LatchSize + 0.4 mm"
equation "d172 = LatchSize + 1.4 mm"
equation "HingeSize = 15 mm"
equation "LatchSize = 20 mm"
equation "d188 = LatchSize"
equation "d191 = LatchSize - 3 mm"
equation "d194 = LatchSize - 2 mm"
equation "d199 = LatchSize - 3 mm"
equation "d210 = LatchSize + 8 mm"
equation "d213 = LatchSize + 0.4 mm"
equation "d216 = LatchSize - 2.6 mm"
equation "d226 = LatchSize - 2.2 mm"
equation "d257 = -Height + 7 mm"
equation "d261 = -Height + 1 mm"
equation "d279 = Height - 8 mm"
equation "RowSectionDistance = ( Width - 4 mm ) / Rows"
equation "ColumnSectionDistance = ( Length - 4 mm ) / Columns"
equation "d283 = Columns"
equation "d285 = ColumnSectionDistance"
equation "d288 = Height - 8 mm"
equation "d290 = Rows"
equation "d292 = RowSectionDistance"
equation "Rows = 1"
equation "Columns = 1"
equation "d324 = HingePosition"
equation "d325 = HingeSize + 2.4 mm"
equation "d337 = Width + 3.2 mm"
equation "SlotWidth = 80 mm"
equation "SlotLength = 80 mm"
equation "SlotHeight = 30 mm"
equation "d342 = Height - 4 mm"
equation "d343 = Height - 24 mm"
equation "d352 = Height - 15 mm"
equation "d356 = Width + 3.2 mm"
equation "LogoWidth = 50 mm"
equation "d371 = LogoWidth / 50 mm"
named bodies: "Box", "Lid", "Body8 (1)", "Body9 (1)", "Body12 (1)", "Body14 (1)", "Body16 (1)", "Body18 (1)", "Body20 (1)", "Body25 (1)", "Body27 (1)", "Body29 (1)", "Body30 (1)", "Body30 (2)", "Body31 (1)", "Body31 (1) (1)", "Latch", "Lid Hinge"
